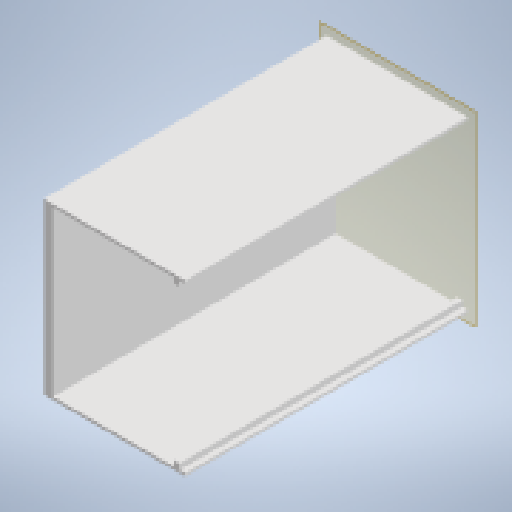
# Autodesk Inventor part: ForwardSection1
Saved by Autodesk Inventor 2026 (Build 300175050, 175E)
## iProperties
Created: 2025-08-01
Part Number: ForwardSection1
Material: Plastic, Opaque White
Document SubType Name: Modeling
Designer: Cupri
Density: 0.952 g/cm^3
Appearance: Smooth - White
Author: Cupri
Autodesk Inventor part; units mm, degrees
ref_plane "YZ Plane" through (0, 0, 0) normal (1, 0, 0) x (0, 1, 0)
ref_plane "Work Plane1" through (0, 0, 0) normal (0, 0, 1) x (1, 0, 0)
sketch "Sketch1" plane through (0, 0, 0) normal (0, 0, 1) x (1, 0, 0)
  line L0 (0, -150) -> (-125.0759, -150) projected
  line L1 (0, 0) -> (0, -150) projected
  line L2 (-125.0759, 0) -> (0, 0) projected
  line L3 (-125.0759, 0) -> (-125.0759, -150) projected
  line L4 (-5, -147.5) -> (-117.0759, -147.5) projected
  line L5 (-117.0759, -147.5) -> (-117.0759, -2.5) projected
  line L6 (-117.0759, -2.5) -> (-5, -2.5) projected
  line L7 (-5, -2.5) -> (-5, -147.5) projected
  line L8 (0, -150) -> (-125.0759, -150) projected
  line L9 (0, 0) -> (0, -150) projected
  line L10 (-125.0759, 0) -> (0, 0) projected
  line L11 (-125.0759, 0) -> (-125.0759, -150) projected
  line L12 (-5, -147.5) -> (-117.0759, -147.5) projected
  line L13 (-117.0759, -147.5) -> (-117.0759, -2.5) projected
  line L14 (-117.0759, -2.5) -> (-5, -2.5) projected
  line L15 (-5, -2.5) -> (-5, -147.5) projected
  line L16 (-5, -2.5) -> (0, -2.5)
  line L17 (-5, -147.5) -> (0, -147.5)
  line L18 (-5, -2.5) -> (-10, -2.5)
  line L19 (-10, -2.5) -> (-10, -7.5)
  line L20 (-10, -7.5) -> (-5, -7.5)
  line L21 (-5, -7.5) -> (-5, -2.5)
  line L22 (-5, -147.5) -> (-10, -147.5)
  line L23 (-10, -147.5) -> (-10, -142.5)
  line L24 (-10, -142.5) -> (-5, -142.5)
  line L25 (-5, -142.5) -> (-5, -147.5)
  dimension "d2" = 5
  dimension "d3" = 5
  dimension "d4" = 5
  dimension "d5" = 5
  constraints: 20 end point, 4 parallel, 4 perpendicular, 2 horizontal, 2 point on line
  measures "d2" distance of L20.end L19.end
  measures "d3" distance of L19.end L18.end
  measures "d4" distance of L23.end L24.end
  measures "d5" distance of L22.end L23.end
extrude "Extrusion1" add sketch "Sketch1" along normal blind 250 contours L0 L3 L2 L1 L16 L6 L5 L4 L17 | L4 L23 L24 L7 | L7 L20 L19 L6
sketch "Sketch2" plane through (0, 0, 250) normal (0, 0, 1) x (1, 0, 0)
  line L0 (-5, -2.5) -> (-2, -2.5)
  line L1 (-2, -2.5) -> (-2, -7.5)
  line L2 (0, -2.5) -> (-2, -2.5)
  line L3 (-2, -2.5) -> (-2, -7.5)
  line L4 (-2, -7.5) -> (0, -7.5)
  line L5 (0, -7.5) -> (0, -2.5)
  line L6 (-117.0759, -147.5) -> (-117.0759, -2.5) projected
  line L7 (-117.0759, -75) -> (40.0034, -75) construction
  line L8 (-5, -147.5) -> (-2, -147.5)
  line L9 (-2, -147.5) -> (-2, -142.5)
  line L10 (0, -147.5) -> (-2, -147.5)
  line L11 (-2, -147.5) -> (-2, -142.5)
  line L12 (-2, -142.5) -> (0, -142.5)
  line L13 (0, -142.5) -> (0, -147.5)
  point P0 (0, 0)
  constraints: 26 end point, 6 symmetric about line, 3 horizontal, 2 parallel, 2 perpendicular, 1 midpoint
ref_plane "Work Plane2" through (-125.0759, -150, 0) normal (0, 0, 1) x (1, 0, 0)
extrude "Extrusion2" add sketch "Sketch2" against normal up to surface (250 mm away)
fillet "Fillet1" radius 2 2 edges at (-5, -142.5, 125) (-5, -7.5, 125)
sketch "Sketch3" plane through (0, 0, 250) normal (0, 0, 1) x (1, 0, 0)
  line L0 (0, -7.5) -> (0, 0) projected
  line L1 (0, -7.5) -> (-2, -7.5)
  line L2 (-5, -7.5) -> (-5, -142.5)
  line L3 (-2, -142.5) -> (0, -142.5)
  line L4 (0, -142.5) -> (0, -7.5)
  line L5 (-2, -147.5) -> (-2, -142.5) projected
  line L6 (-2, -147.5) -> (-5, -147.5)
  line L7 (-5, -147.5) -> (-5, -142.5)
  line L8 (-2, -142.5) -> (-2, -147.5)
  line L9 (-5, -2.5) -> (-2, -2.5) projected
  line L10 (-2, -2.5) -> (-5, -2.5)
  line L11 (-5, -2.5) -> (-5, -7.5)
  line L12 (-2, -7.5) -> (-2, -2.5)
  line L13 (-2, -2.5) -> (-2, -7.5) projected
  line L14 (-2, -2.7) -> (-5, -2.7)
  line L15 (-2, -147.3) -> (-5, -147.3)
  dimension "d10" = 0.2
  dimension "d11" = 0.2
  constraints: 24 end point, 5 perpendicular, 4 parallel, 4 point on line, 3 horizontal
  measures "d10" distance between parallel lines of L9 L14
  measures "d11" distance between parallel lines of L6 L15
ref_plane "Work Plane3" through (-125.0759, -150, 0) normal (0, 0, 1) x (1, 0, 0)
body "Solid1"
